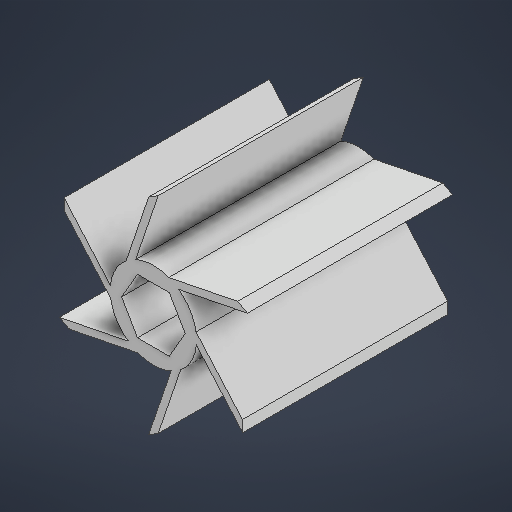
# Autodesk Inventor part: Spiral 2
Saved by Autodesk Inventor 2026.1 (Build 301233000, 233)
## iProperties
Created: 2025-11-03
Part Number: Spiral 2
Material: Generic
Document SubType Name: Modeling
Designer: randy
Density: 1 g/cm^3
Appearance: Default
Author: randy
Autodesk Inventor part; units mm, degrees
ref_plane "YZ Plane" through (0, 0, 0) normal (1, 0, 0) x (0, 1, 0)
ref_plane "XZ Plane" through (0, 0, 0) normal (0, 1, 0) x (-1, 0, 0)
ref_plane "XY Plane" through (0, 0, 0) normal (0, 0, 1) x (1, 0, 0)
sketch "Sketch1" plane through (0, 0, 0) normal (0, 0, 1) x (1, 0, 0)
  circle A0 centre (0, 0) radius 10.16
  circle A1 centre (0, 0) radius 8.5725
  line L0 (-4.1708, 9.2644) -> (1.118, 24.9044)
  line L1 (1.118, 24.9044) -> (-1.118, 23.5253)
  line L2 (-1.118, 23.5253) -> (-6.4068, 7.8853)
  line L3 (-7.479, 0) -> (-3.7395, 6.477)
  line L4 (-3.7395, 6.477) -> (3.7395, 6.477)
  line L5 (3.7395, 6.477) -> (7.479, 0)
  line L6 (7.479, 0) -> (3.7395, -6.477)
  line L7 (3.7395, -6.477) -> (-3.7395, -6.477)
  line L8 (-3.7395, -6.477) -> (-7.479, 0)
  line L9 (-10.1087, 1.0202) -> (-21.0088, 13.4204)
  line L10 (-21.0088, 13.4204) -> (-20.9325, 10.7944)
  line L11 (-20.9325, 10.7944) -> (-10.0323, -1.6058)
  line L12 (-5.9378, -8.2443) -> (-22.1269, -11.484)
  line L13 (-22.1269, -11.484) -> (-19.8145, -12.7309)
  line L14 (-19.8145, -12.7309) -> (-3.6254, -9.4911)
  line L15 (4.1708, -9.2644) -> (-1.118, -24.9044)
  line L16 (-1.118, -24.9044) -> (1.118, -23.5253)
  line L17 (1.118, -23.5253) -> (6.4068, -7.8853)
  line L18 (10.1087, -1.0202) -> (21.0088, -13.4204)
  line L19 (21.0088, -13.4204) -> (20.9325, -10.7944)
  line L20 (20.9325, -10.7944) -> (10.0323, 1.6058)
  line L21 (5.9378, 8.2443) -> (22.1269, 11.484)
  line L22 (22.1269, 11.484) -> (19.8145, 12.7309)
  line L23 (19.8145, 12.7309) -> (3.6254, 9.4911)
  point P0 (0, 24.2148)
  point P1 (-20.9707, 12.1074)
  point P2 (-20.9707, -12.1074)
  point P3 (0, -24.2148)
  point P4 (20.9707, -12.1074)
  point P5 (20.9707, 12.1074)
  point P6 (-10.0323, -1.6058)
  point P7 (-10.1087, 1.0202)
  point P8 (6.4068, -7.8853)
  point P9 (4.1708, -9.2644)
  point P10 (10.1087, -1.0202)
  point P11 (-3.6254, -9.4911)
  point P12 (-5.9378, -8.2443)
  point P13 (3.6254, 9.4911)
  point P14 (5.9378, 8.2443)
  dimension "d0" = 20.32
  dimension "d1" = 1.5875
  dimension "d7" = 1.6764
  dimension "d13" = 16.51
  dimension "d17" = 12.954
  dimension "d20" = 360
  dimension "d22" = 6.9188
  constraints: 48 end point, 2 centre point, 2 coincident, 2 parallel, 2 point on circle, 1 horizontal, 1 midpoint, 1 vertical alignment, 62 other
  measures "d0" diameter of A0
  measures "d1" radial gap between concentric circles of A0 A1
  measures "d7" distance between parallel lines of L2 L0
  measures "d13" distance of L0.start L0.end
  measures "d17" distance between parallel lines of L7 L4
  measures "d22" distance from line of A1.centre L0
extrude "Extrusion1" add sketch "Sketch1" along normal mid plane 48.26 contours A0 | A0 L20 L19 L18 | A0 L23 L22 L21 | L17 L16 L15 A0 | A0 L2 L1 L0 | L14 L13 L12 A0 | A0 L11 L10 L9 | A1
body "Solid1"
